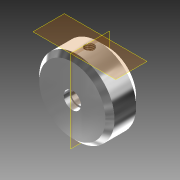
# Autodesk Inventor part: D-041
Saved by Autodesk Inventor 2015 (Build 190159000, 159)
## iProperties
Company: MARCHA TECHNOLOGY
Created: 2013-10-24
Part Number: D-041
Document SubType Name: Modeling
Designer: O.Martin
Density: 1 g/cm^3
Mass: 9.3992 g
Surface Area: 30.922 cm^2
Volume: 9.3992 cm^3
Project: WITBOXprinter_K01
Description: RUEDA CONTROL
Stock Number: 28655
Material: Generic
Appearance: Chrome - Polished Black
Author: O.Martin
Autodesk Inventor part; units mm, degrees
ref_plane "XZ Plane" through (0, 0, 0) normal (0, 1, 0) x (-1, 0, 0)
sketch "Boceto1" plane through (0, 0, 0) normal (0, 0, 1) x (1, 0, 0)
  line L0 (0, 15.5) -> (0, 0)
  line L1 (0, 0) -> (-16.5, 0)
  line L2 (-16.5, 0) -> (-16.5, 15.5)
  line L3 (-16.5, 15.5) -> (0, 15.5)
  circle A0 centre (-7, 19.5) radius 6
  line L4 (-7, 13.5) -> (-7, 25.5)
  line L5 (-3, 0) -> (-3, 14.5)
  line L6 (-3, 14.5) -> (0, 14.5)
  line L7 (-3, 0) -> (-3.75, 0)
  line L8 (-3.75, 0) -> (-3.75, 2.5)
  line L9 (-3.75, 2.5) -> (-3, 2.5)
  line L10 (-3, 2.5) -> (-3, 0)
  point P0 (-7, 19.5)
  dimension "d0" = 33
  dimension "d4" = 12
  dimension "d5" = 7
  dimension "d6" = 2
  dimension "d13" = 15.5
  dimension "d38" = 6
  dimension "d47" = 1
  dimension "d49" = 7.5
  dimension "d50" = 2.5
  constraints: 22 end point, 3 parallel, 2 coincident, 2 horizontal, 2 perpendicular, 2 point on circle, 2 point on line, 1 centre point, 1 midpoint, 1 vertical
  measures "d0" diameter of L2 L0
  measures "d4" diameter of A0
  measures "d5" distance between parallel lines of L0 L4
  measures "d6" distance from line of L3 L4.start
  measures "d13" distance of L1.end L2.end
  measures "d38" diameter of L5 L0
  measures "d47" distance between parallel lines of L3 L6
  measures "d49" diameter of L8 L0
  measures "d50" distance of L7.end L8.end
revolve "Revolución1" add sketch "Boceto1" angle 360 about axis through (0, 15.5, 0) along (0, -1, 0) picked at (-4.3297, 15.2182) picked at (-9.6703, 15.2182) contours L0 L6 L5 L9 L8 L1 L2 L3 A0 | A0 L4 L3 | L4 A0 L3
revolve "Revolución2" cut sketch "Boceto1" angle 360 about axis through (-7, 13.5, 0) along (0, 1, 0) picked at (-9.6703, 15.2182) picked at (-7.4561, 22.114) contours L4 A0 L3 | L3 A0 L4
chamfer "Chaflán1" distance 4 angle 45 1 edges at (16.5, 15.5, 0)
ref_plane "Plano de trabajo1" through (0, 7.75, 16.5) normal (0, 0, 1) x (1, 0, 0)
sketch "Boceto2" plane through (0, 7.75, 16.5) normal (0, 0, 1) x (1, 0, 0)
  line L0 (16.5, -7.75) -> (-16.5, -7.75) projected
  line L1 (3, 6.75) -> (-3, 6.75) projected
  point P0 (0, -0.25)
  point P1 (0, -7.75)
  dimension "d48" = 7.5
  constraints: 1 midpoint, 1 vertical alignment
  measures "d48" distance from line of point (0, -0.25) L0
hole "Agujero2" at (0, 7.5, 16.5) direction (0, 0, -1) diameter 4.134 depth 15 tip angle 118 thread size "M5x0.8" class "6H" standard "ISO Metric profile"
chamfer "Chaflán2" distance 2 angle 45 1 edges at (16.5, 0, 0)
body "Solid1"
